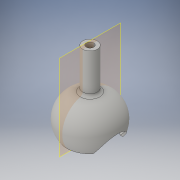
# Autodesk Inventor part: mcdave caster
Saved by Autodesk Inventor 2016 (Build 200138000, 138)
## iProperties
Created: 2016-10-19
Part Number: mcdave caster
Material: Generic
Document SubType Name: Modeling
Designer: ClenoR
Density: 1 g/cm^3
Appearance: Default
Sheet Metal Rule: Default
Author: ClenoR
Autodesk Inventor part; units mm, degrees
ref_plane "XZ Plane" through (0, 0, 0) normal (0, 1, 0) x (-1, 0, 0)
ref_plane "XY Plane" through (0, 0, 0) normal (0, 0, 1) x (1, 0, 0)
sketch "Sketch1" plane through (0, 0, 0) normal (0, 0, 1) x (1, 0, 0)
  arc A0 (0, 15.3683) -> (-19.6378, -9.7289) centre (-2.7904, -2.6799) ccw
  arc A1 (-5.842, 16.6129) -> (-21.0429, -9.6347) centre (-2.7904, -2.6799) ccw
  line L0 (0, 51.5125) -> (-5.842, 51.5125)
  line L1 (-5.842, 51.5125) -> (-5.842, 16.6129)
  line L2 (0, 15.3683) -> (0, 51.5125)
  arc A2 (0, 15.3683) -> (-17.0727, -14.0614) centre (-2.7904, -2.6799) ccw
  arc A3 (0, 16.6524) -> (-18.6644, -14.0614) centre (-2.7904, -2.6799) ccw
  line L3 (-18.6644, -14.0614) -> (-17.0727, -14.0614)
  dimension "d3" = 1.27
  dimension "d5" = 34.8996
  dimension "d6" = 18.2626
  dimension "d7" = 5.842
  dimension "d9" = 36.1442
  constraints: 10 point on circle, 8 end point, 4 centre point, 3 coincident, 2 horizontal, 1 perpendicular, 1 point on line, 1 vertical
  measures "d3" radial gap between concentric circles of A1 A0
  measures "d5" distance of L0.end L1.end
  measures "d6" radius of A0
  measures "d7" distance of L0.start L0.end
  measures "d9" distance from line of L2.start L0
revolve "Revolution1" add sketch "Sketch1" angle 360 about axis through (0, 15.3683, 0) along (0, 1, 0)
sketch "Sketch4" plane through (0, 51.5125, 0) normal (0, 1, 0) x (1, 0, 0)
  circle A0 centre (0, 0) radius 5.842 projected
  circle A1 centre (0, 0) radius 2.9972
  point P0 (0, 0)
  dimension "d21" = 5.9944
  constraints: 1 centre point, 1 coincident
  measures "d21" diameter of A1
extrude "Cut1" cut sketch "Sketch4" against normal blind 3.048 contours A0 | A1
sketch "Sketch5" plane through (0, 0, 0) normal (1, 0, 0) x (0, 1, 0)
  line L0 (3.3342, -12.2505) -> (3.3342, 12.2505) projected
  circle A0 centre (3.3342, 0) radius 7.99
  point P0 (0, 0)
  constraints: 1 centre point, 1 midpoint
extrude "Extrusion3" cut sketch "Sketch5" along normal mid plane 25.4
sketch "Sketch6" plane through (0, 48.4645, 0) normal (0, 1, 0) x (1, 0, 0)
  circle A0 centre (0, 0) radius 2.9972
  point P0 (0, 0)
  dimension "d22" = 5.9944
  constraints: 1 centre point, 1 coincident
  measures "d22" diameter of A0
extrude "Extrusion4" cut sketch "Sketch6" against normal blind 12.7
sketch "Sketch7" plane through (-12.7, 0, 0) normal (1, 0, 0) x (0, 0, -1)
  circle A0 centre (0, 6.8594) radius 3.3582
  point P0 (0, 0)
  constraints: 1 centre point
extrude "Extrusion5" [suppressed]
sketch "Sketch8" plane through (-12.7, 0, 0) normal (1, 0, 0) x (0, 0, -1)
  circle A0 centre (0.7643, 6.3089) radius 4.4927
  point P0 (0, 0)
  constraints: 1 centre point
extrude "Extrusion6" [suppressed]
sketch "Sketch9" plane through (12.7, 0, 0) normal (-1, 0, 0) x (0, 0, 1)
  circle A0 centre (0, 6.8376) radius 3.6987
  point P0 (0, 0)
  constraints: 1 centre point
extrude "Extrusion7" [suppressed]
fillet "Fillet1" radius 2.54 1 edges at (5.842, 16.6129, 0)
sketch "Sketch10" plane through (0, 0, 0) normal (1, 0, 0) x (0, 1, 0)
  line L0 (-14.0614, -17.0727) -> (-14.0614, 17.0727) projected
  circle A0 centre (-14.0614, 0) radius 11.9423
  point P0 (0, 0)
  constraints: 1 centre point, 1 midpoint
extrude "Extrusion8" cut sketch "Sketch10" against normal blind 25.4
sketch "Sketch11" plane through (0, 0, 0) normal (1, 0, 0) x (0, 1, 0)
  line L0 (-14.0614, -17.0727) -> (-14.0614, 17.0727) projected
  circle A0 centre (-14.0614, 0) radius 11.938
  point P0 (0, 0)
  point P1 (-14.0614, 11.9423)
  point P2 (-14.0614, -11.9423)
  dimension "d34" = 23.876
  constraints: 1 centre point, 1 midpoint
  measures "d34" diameter of A0
extrude "Extrusion9" cut sketch "Sketch11" along normal blind 25.4
equation "\"d17\" = Thickness"
equation "\"BendRadius\" = Thickness"
equation "\"BendReliefWidth\" = Thickness"
equation "\"BendReliefDepth\" = 0.5 * Thickness"
equation "\"CornerReliefSize\" = 4 * Thickness"
equation "\"MinimumRemnant\" = 2 * Thickness"
equation "\"TransitionRadius\" = BendRadius"
equation "\"JacobiRadiusSize\" = Thickness"
equation "\"GapSize\" = Thickness"
equation "\"Thickness\" = 3.048"
body "Solid1"
